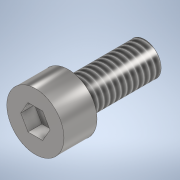
# Autodesk Inventor part: UC-2606
Saved by Autodesk Inventor 2022 (Build 260153000, 153)
## iProperties
Part Number: UC-2606
Material: ステンレス鋼 AISI 304
Document SubType Name: Modeling
Designer: Masato Kubotera
Density: 6.37146 g/cm^3
Appearance: 半つや出し
Mass: 0.347 g
Surface Area: 1.13586 cm^2
Volume: 0.0544616 cm^3
Description: ReadyMade
Catalog Web Link: https://wilco.jp/products/F/FC-EB.html#page3
Author: Masato Kubotera
Comments: Width across flats : 1.5
Autodesk Inventor part; units mm, degrees
ref_plane "YZ Plane" through (0, 0, 0) normal (1, 0, 0) x (0, 1, 0)
ref_plane "XZ Plane" through (0, 0, 0) normal (0, 1, 0) x (-1, 0, 0)
ref_plane "XY Plane" through (0, 0, 0) normal (0, 0, 1) x (1, 0, 0)
sketch "スケッチ1" plane through (0, 0, 0) normal (1, 0, 0) x (0, 1, 0)
  line L0 (0, 8.6) -> (0, 0)
  line L1 (0, 0) -> (2.25, 0)
  line L2 (2.25, 0) -> (2.25, 2.6)
  line L3 (2.25, 2.6) -> (1.3, 2.6)
  line L4 (1.3, 2.6) -> (1.3, 8.6)
  line L5 (1.3, 8.6) -> (0, 8.6)
  dimension "d2" = 2.6
  dimension "d10" = 6
  dimension "d11" = 2.6
  dimension "d12" = 4.5
  constraints: 12 end point, 5 perpendicular, 1 vertical
  measures "d2" distance of L1.end L2.end
  measures "d10" distance of L3.end L4.end
  measures "d11" diameter of L4 L0
  measures "d12" diameter of L2 L0
revolve "回転1" add sketch "スケッチ1" angle 360 about axis through (0, 0, 8.6) along (0, 0, -1)
thread "ねじ1" size "M2.6x0.45" class "6g" standard "ANSI Metric M Profile" full length
sketch "スケッチ2" plane through (0, 0, 0) normal (0, 0, -1) x (-1, 0, 0)
  line L0 (0, 1.1547) -> (1, 0.5774)
  line L1 (1, 0.5774) -> (1, -0.5774)
  line L2 (1, -0.5774) -> (0, -1.1547)
  line L3 (0, -1.1547) -> (-1, -0.5774)
  line L4 (-1, -0.5774) -> (-1, 0.5774)
  line L5 (-1, 0.5774) -> (0, 1.1547)
  circle A0 centre (0, 0) radius 2.25 projected
  line L6 (0, 2.25) -> (0, -2.25) construction
  point P0 (0, 0)
  dimension "d7" = 2
  constraints: 14 end point, 2 point on circle, 1 coincident, 1 midpoint, 1 point on line, 1 vertical, 13 other
  measures "d7" distance between parallel lines of L1 L4
extrude "押し出し1" cut sketch "スケッチ2" against normal blind 1.1 contours L0 L1 L2 L3 L4 L5
